Autodesk Inventor part; units mm, degrees
(part 5 of 18)
  spline S48 degree 3 poles (-10072.1223, -10008.9292) (-10072.1359, -10008.9311) (-10072.1627, -10008.9349) (-10072.2009, -10008.9472) (-10072.2359, -10008.9639) (-10072.2669, -10008.9851) (-10072.2932, -10009.0101) (-10072.314, -10009.0387) (-10072.326, -10009.0652) (-10072.3319, -10009.0875) (-10072.3344, -10009.1048) (-10072.335, -10009.1227) (-10072.3334, -10009.141) (-10072.3297, -10009.1596) (-10072.3239, -10009.178) (-10072.3161, -10009.1959) (-10072.3033, -10009.2187) (-10072.2831, -10009.2451) (-10072.2535, -10009.2724) (-10072.2194, -10009.2948) (-10072.1818, -10009.3124) (-10072.1549, -10009.3189) (-10072.1414, -10009.3222) knots 0 0 0 0 0.067054 0.132171 0.195214 0.256087 0.314845 0.371833 0.427831 0.455897 0.484265 0.513193 0.542966 0.573892 0.605563 0.637232 0.669027 0.733247 0.798614 0.865047 0.932273 1 1 1 1
  spline S49 degree 3 poles (-10072.1484, -10009.347) (-10072.1552, -10009.3452) (-10072.1688, -10009.3417) (-10072.1951, -10009.331) (-10072.2261, -10009.3129) (-10072.2593, -10009.2847) (-10072.288, -10009.2513) (-10072.3115, -10009.2138) (-10072.3291, -10009.1734) (-10072.3399, -10009.1312) (-10072.3427, -10009.0953) (-10072.3408, -10009.067) (-10072.3371, -10009.0462) (-10072.3313, -10009.0261) (-10072.3234, -10009.0072) (-10072.3137, -10008.9897) (-10072.2986, -10008.9682) (-10072.2756, -10008.9447) (-10072.2429, -10008.9219) (-10072.2064, -10008.9046) (-10072.1671, -10008.8921) (-10072.1397, -10008.8879) (-10072.1259, -10008.8858) knots 0 0 0 0 0.031337 0.062781 0.126297 0.190936 0.256459 0.32232 0.387875 0.452577 0.516183 0.547678 0.57907 0.610325 0.640706 0.670386 0.69965 0.757762 0.816478 0.876441 0.937726 1 1 1 1
  spline S50 degree 3 poles (-10072.0136, -10008.8866) (-10072.0011, -10008.8889) (-10071.9769, -10008.8935) (-10071.9435, -10008.9084) (-10071.9145, -10008.9285) (-10071.8903, -10008.9537) (-10071.8713, -10008.9835) (-10071.8579, -10009.0174) (-10071.8502, -10009.0548) (-10071.8486, -10009.0953) (-10071.8534, -10009.1379) (-10071.8643, -10009.1807) (-10071.8813, -10009.2213) (-10071.9037, -10009.258) (-10071.9309, -10009.2899) (-10071.9573, -10009.312) (-10071.9802, -10009.3264) (-10071.9982, -10009.3354) (-10072.017, -10009.3428) (-10072.03, -10009.3461) (-10072.0365, -10009.3477) knots 0 0 0 0 0.060227 0.117303 0.172542 0.227241 0.282631 0.339845 0.399897 0.463695 0.532058 0.603464 0.673189 0.741116 0.807351 0.872143 0.90418 0.93608 0.967968 1 1 1 1
  spline S51 degree 3 poles (-10072.0296, -10009.3229) (-10072.0263, -10009.3223) (-10072.0197, -10009.3209) (-10072.01, -10009.3183) (-10072.0005, -10009.3153) (-10071.9882, -10009.3107) (-10071.9732, -10009.3038) (-10071.9562, -10009.294) (-10071.9401, -10009.2827) (-10071.9251, -10009.2702) (-10071.911, -10009.2565) (-10071.9026, -10009.2466) (-10071.8984, -10009.2416) knots 0 0 0 0 0.06406 0.127639 0.190828 0.253706 0.37877 0.503307 0.627605 0.751814 0.875967 1 1 1 1
  spline S52 degree 3 poles (-10071.8529, -10009.0281) (-10071.8545, -10009.0246) (-10071.8575, -10009.0175) (-10071.8632, -10009.0076) (-10071.8696, -10008.9982) (-10071.8767, -10008.9895) (-10071.8845, -10008.9813) (-10071.8931, -10008.9738) (-10071.9022, -10008.9668) (-10071.9121, -10008.9605) (-10071.9225, -10008.9547) (-10071.9335, -10008.9495) (-10071.945, -10008.9449) (-10071.9571, -10008.9408) (-10071.9697, -10008.9373) (-10071.9827, -10008.9343) (-10071.9962, -10008.9318) (-10072.0053, -10008.9306) (-10072.01, -10008.93) knots 0 0 0 0 0.059633 0.118254 0.176262 0.234034 0.291919 0.350232 0.409251 0.469215 0.530325 0.592744 0.656603 0.721998 0.789001 0.857656 0.927988 1 1 1 1
  ellipse E575 centre (-10070.5168, -10009.0175) end of major axis (-10070.2676, -10008.9967) minor radius 0.1227 (-10070.4266, -10008.897) -> (-10070.5389, -10008.8963) ccw
  ellipse E576 centre (-10070.5132, -10009.0609) end of major axis (-10070.7623, -10009.0817) minor radius 0.1227 (-10070.423, -10008.9404) -> (-10070.5353, -10008.9397) ccw
  ellipse E577 centre (-10072.1038, -10009.007) end of major axis (-10071.8546, -10008.9862) minor radius 0.1227 (-10072.0136, -10008.8866) -> (-10072.1259, -10008.8858) ccw
  ellipse E578 centre (-10072.1001, -10009.0504) end of major axis (-10072.3493, -10009.0712) minor radius 0.1227 (-10072.01, -10008.93) -> (-10072.1223, -10008.9292) ccw
  ellipse E579 centre (-10070.5162, -10009.1216) end of major axis (-10070.2755, -10009.1894) minor radius 0.2142 (-10070.5544, -10009.3326) -> (-10070.4426, -10009.3334) ccw
  ellipse E580 centre (-10072.1031, -10009.1112) end of major axis (-10071.8625, -10009.1789) minor radius 0.2142 (-10072.1414, -10009.3222) -> (-10072.0296, -10009.3229) ccw
  ellipse E581 centre (-10070.2084, -10009.1917) end of major axis (-10070.2065, -10008.9037) minor radius 0.0453 (-10070.2293, -10008.9417) -> (-10070.2487, -10009.3347) ccw
  ellipse E582 centre (-10070.2084, -10009.1917) end of major axis (-10070.2107, -10009.5297) minor radius 0.0531 (-10070.2329, -10008.8983) -> (-10070.2557, -10009.3595) ccw
  ellipse E583 centre (-10072.2951, -10009.178) end of major axis (-10072.2973, -10009.516) minor radius 0.0531 (-10072.3196, -10008.8846) -> (-10072.3423, -10009.3457) ccw
  line L687 (-10070.1881, -10008.7391) -> (-10070.2329, -10008.8983)
  line L688 (-10072.3196, -10008.8846) -> (-10072.3149, -10008.8679)
  line L689 (-10072.3105, -10008.8522) -> (-10072.3069, -10008.8393)
  line L690 (-10070.1841, -10008.7811) -> (-10070.2293, -10008.9417)
  line L691 (-10072.2871, -10029.6576) -> (-10072.2821, -10029.5511)
  ellipse E584 centre (-10072.6143, -10008.6378) end of major axis (-10072.3161, -10008.7222) minor radius 0.2558 (-10072.3088, -10008.6455) -> (-10072.3104, -10008.6316) ccw
  line L692 (-10072.3104, -10008.6316) -> (-10072.2913, -10008.5643)
  line L693 (-10072.3046, -10008.6951) -> (-10072.3088, -10008.6455)
  arc A6 (-10072.145, -10030.9182) -> (-10072.0351, -10030.8171) centre (-10072.2938, -10030.6462) ccw
  ellipse E585 centre (-10072.1984, -10008.6427) end of major axis (-10072.1761, -10008.2008) minor radius 0.0791 (-10072.2594, -10008.4435) -> (-10072.261, -10008.4555) ccw
  arc A7 (-10072.0403, -10007.364) -> (-10072.1626, -10007.2386) centre (-10072.3143, -10007.509) ccw
  ellipse E586 centre (-10072.6346, -10029.3671) end of major axis (-10072.3396, -10029.2718) minor radius 0.274 (-10072.3299, -10029.3798) -> (-10072.3284, -10029.365) ccw
  line L694 (-10072.325, -10029.3952) -> (-10072.3299, -10029.3798)
  line L695 (-10072.3284, -10029.365) -> (-10072.3184, -10029.2255)
  ellipse E587 centre (-10072.6677, -10009.4402) end of major axis (-10072.3588, -10009.4144) minor radius 0.1522 (-10072.3645, -10009.4509) -> (-10072.3616, -10009.4422) ccw
  line L696 (-10072.3562, -10009.5506) -> (-10072.3645, -10009.4509)
  ellipse E588 centre (-10072.6401, -10008.8765) end of major axis (-10072.3417, -10008.9605) minor radius 0.2656 (-10072.3339, -10008.8785) -> (-10072.3356, -10008.8642) ccw
  line L697 (-10072.3356, -10008.8642) -> (-10072.3215, -10008.8144)
  line L698 (-10072.3296, -10008.93) -> (-10072.3339, -10008.8785)
  line L699 (-10072.3616, -10009.4422) -> (-10072.3467, -10009.3895)
  ellipse E589 centre (-10072.2686, -10009.2994) end of major axis (-10072.2657, -10008.8569) minor radius 0.0696 (-10072.3276, -10009.0793) -> (-10072.3299, -10009.1054) ccw
  arc A8 (-10070.2041, -10029.4572) -> (-10070.1804, -10029.5914) centre (-10069.8944, -10029.4717) ccw
  line L700 (-10070.1804, -10029.5914) -> (-10070.1612, -10029.6371)
  line L701 (-10070.1889, -10029.1314) -> (-10070.2041, -10029.4572)
  arc A9 (-10070.1531, -10029.8637) -> (-10070.147, -10029.8789) centre (-10069.8629, -10029.7549) ccw
  arc A10 (-10070.1727, -10029.7444) -> (-10070.1621, -10029.8358) centre (-10069.8629, -10029.7549) ccw
  line L702 (-10070.147, -10029.8789) -> (-10070.1076, -10029.9691)
  line L703 (-10070.1685, -10029.6198) -> (-10070.1727, -10029.7444)
  arc A11 (-10064.8037, -10028.4984) -> (-10064.8044, -10028.4963) centre (-10065.9342, -10028.9009) ccw
  line L704 (-10065.7396, -10009.9143) -> (-10064.7957, -10009.8155)
  line L705 (-10065.7396, -10028.2797) -> (-10064.7957, -10028.3785)
  arc A12 (-10064.8044, -10009.6977) -> (-10064.8037, -10009.6956) centre (-10065.9342, -10009.2931) ccw
  arc A13 (-10061.9634, -10012.6939) -> (-10061.989, -10012.5783) centre (-10063.1464, -10012.895) ccw
  line L706 (-10063.2547, -10012.3915) -> (-10063.1965, -10012.3786)
  arc A14 (-10061.989, -10025.6156) -> (-10061.9634, -10025.5) centre (-10063.1464, -10025.299) ccw
  line L707 (-10063.2547, -10025.8025) -> (-10063.1965, -10025.8154)
  arc A15 (-10062.9803, -10029.3632) -> (-10062.946, -10028.8732) centre (-10064.1349, -10029.0362) ccw
  line L708 (-10075.6049, -10030.1318) -> (-10075.4175, -10030.1223)
  line L709 (-10074.3953, -10030.0706) -> (-10074.2526, -10030.0634)
  line L710 (-10068.1084, -10029.7528) -> (-10065.7939, -10029.6358)
  line L711 (-10064.718, -10029.5814) -> (-10064.0364, -10029.5469)
  arc A16 (-10062.0783, -10026.4492) -> (-10062.0721, -10026.3309) centre (-10063.2721, -10026.3271) ccw
  line L712 (-10063.2578, -10025.8122) -> (-10063.1965, -10025.8154)
  line L713 (-10064.0581, -10026.8015) -> (-10063.1016, -10026.8518)
  line L714 (-10064.2047, -10013.5891) -> (-10064.1279, -10013.5729)
  arc A17 (-10061.7588, -10010.2049) -> (-10061.7925, -10009.906) centre (-10062.9587, -10010.1889) ccw
  line L715 (-10063.7731, -10009.7624) -> (-10062.8324, -10009.6564)
  line L716 (-10063.6658, -10010.7869) -> (-10062.717, -10010.6799)
  arc A18 (-10061.7925, -10028.288) -> (-10061.7588, -10027.9891) centre (-10062.9587, -10028.0051) ccw
  line L717 (-10063.6658, -10027.4071) -> (-10062.717, -10027.5141)
  line L718 (-10063.7731, -10028.4315) -> (-10062.8324, -10028.5376)
  line L719 (-10064.2047, -10024.6048) -> (-10064.1279, -10024.6211)
  arc A19 (-10062.0721, -10011.8631) -> (-10062.0783, -10011.7448) centre (-10063.2721, -10011.8669) ccw
  line L720 (-10064.0581, -10011.3925) -> (-10063.1016, -10011.3422)
  line L721 (-10063.2578, -10012.3818) -> (-10063.1965, -10012.3786)
  arc A20 (-10062.946, -10009.3208) -> (-10062.9803, -10008.8308) centre (-10064.1349, -10009.1577) ccw
  line L722 (-10075.6049, -10008.0622) -> (-10075.4175, -10008.0717)
  line L723 (-10074.3953, -10008.1234) -> (-10074.285, -10008.1289)
  line L724 (-10068.1392, -10008.4396) -> (-10065.7939, -10008.5582)
  line L725 (-10064.718, -10008.6126) -> (-10064.0364, -10008.6471)
  line L726 (-10075.5477, -10028.2832) -> (-10075.5066, -10028.2829)
  line L727 (-10068.1881, -10028.2347) -> (-10067.699, -10028.2314)
  line L728 (-10068.3069, -10010.1041) -> (-10066.7715, -10009.9541)
  line L729 (-10068.3069, -10028.0898) -> (-10066.7715, -10028.2399)
  line L730 (-10075.5477, -10009.9108) -> (-10075.5066, -10009.9111)
  line L731 (-10068.1987, -10009.9593) -> (-10067.699, -10009.9625)
  ellipse E590 centre (-10081.3091, -10029.2883) end of major axis (-10081.2663, -10030.9877) minor radius 0.2846 (-10081.484, -10030.4742) -> (-10081.2663, -10030.9877) ccw
  line L732 (-10081.1126, -10030.9839) -> (-10081.2663, -10030.9877)
  ellipse E591 centre (-10081.3091, -10008.9057) end of major axis (-10081.2663, -10007.2062) minor radius 0.2846 (-10081.2663, -10007.2062) -> (-10081.484, -10007.7198) ccw
  line L733 (-10081.1126, -10007.2101) -> (-10081.2663, -10007.2062)
  ellipse E592 centre (-10079.4642, -10029.8112) end of major axis (-10079.3783, -10031.5091) minor radius 0.3038 (-10079.6701, -10030.7592) -> (-10079.3783, -10031.5091) ccw
  line L734 (-10079.235, -10031.5018) -> (-10079.3783, -10031.5091)
  ellipse E593 centre (-10079.4642, -10008.3827) end of major axis (-10079.3783, -10006.6849) minor radius 0.3038 (-10079.3783, -10006.6849) -> (-10079.6701, -10007.4347) ccw
  line L735 (-10079.235, -10006.6922) -> (-10079.3783, -10006.6849)
  ellipse E594 centre (-10082.3808, -10011.9965) end of major axis (-10082.5461, -10010.3045) minor radius 0.0977 (-10082.5461, -10010.3045) -> (-10082.5658, -10010.8219) ccw
  line L736 (-10082.2965, -10010.2801) -> (-10082.5461, -10010.3045)
  ellipse E595 centre (-10082.3808, -10026.1975) end of major axis (-10082.5461, -10027.8895) minor radius 0.0977 (-10082.5658, -10027.3721) -> (-10082.5461, -10027.8895) ccw
  line L737 (-10082.2965, -10027.9138) -> (-10082.5461, -10027.8895)
  ellipse E596 centre (-10078.2538, -10029.2113) end of major axis (-10078.2916, -10027.7118) minor radius 0.2511 (-10078.4794, -10028.3382) -> (-10078.5076, -10028.9618) ccw
  ellipse E597 centre (-10078.2538, -10029.2113) end of major axis (-10078.3017, -10027.3119) minor radius 0.3181 (-10078.5573, -10028.33) -> (-10078.4913, -10030.2755) ccw
  ellipse E598 centre (-10081.0135, -10029.2808) end of major axis (-10080.9656, -10031.1802) minor radius 0.3181 (-10081.2919, -10029.9827) -> (-10080.9656, -10031.1802) ccw
  line L738 (-10079.587, -10031.1455) -> (-10080.9656, -10031.1802)
  ellipse E599 centre (-10077.332, -10011.646) end of major axis (-10077.5298, -10009.7564) minor radius 0.0812 (-10077.4803, -10009.9145) -> (-10077.5448, -10009.9731) ccw
  ellipse E600 centre (-10080.1142, -10011.9374) end of major axis (-10080.3121, -10010.0477) minor radius 0.0812 (-10080.3277, -10010.1584) -> (-10080.3141, -10010.5589) ccw
  line L739 (-10077.5298, -10009.7564) -> (-10079.4891, -10009.9615)
  ellipse E601 centre (-10077.332, -10026.5479) end of major axis (-10077.5298, -10028.4376) minor radius 0.0812 (-10077.5448, -10028.2209) -> (-10077.4803, -10028.2794) ccw
  ellipse E602 centre (-10080.1142, -10026.2566) end of major axis (-10080.3121, -10028.1463) minor radius 0.0812 (-10080.3141, -10027.635) -> (-10080.3277, -10028.0355) ccw
  line L740 (-10077.5298, -10028.4376) -> (-10079.4891, -10028.2324)
  ellipse E603 centre (-10078.2538, -10008.9827) end of major axis (-10078.2161, -10007.4832) minor radius 0.2511 (-10078.5076, -10009.2322) -> (-10078.4794, -10009.8558) ccw
  ellipse E604 centre (-10078.2538, -10008.9827) end of major axis (-10078.206, -10007.0833) minor radius 0.3181 (-10078.4913, -10007.9185) -> (-10078.5573, -10009.864) ccw
  ellipse E605 centre (-10081.0135, -10008.9132) end of major axis (-10080.9656, -10007.0138) minor radius 0.3181 (-10080.9656, -10007.0138) -> (-10081.2919, -10008.2112) ccw
  line L741 (-10079.587, -10007.0485) -> (-10080.9656, -10007.0138)
  ellipse E606 centre (-10076.418, -10029.6572) end of major axis (-10076.3422, -10031.1553) minor radius 0.2681 (-10076.6199, -10028.3765) -> (-10076.1967, -10030.8476) ccw
  ellipse E607 centre (-10076.418, -10029.6572) end of major axis (-10076.322, -10031.5548) minor radius 0.3396 (-10076.7301, -10028.364) -> (-10076.0944, -10030.8424) ccw
  ellipse E608 centre (-10079.1694, -10029.7963) end of major axis (-10079.0734, -10031.6939) minor radius 0.3396 (-10079.4714, -10030.3117) -> (-10079.0734, -10031.6939) ccw
  line L742 (-10076.322, -10031.5548) -> (-10079.0734, -10031.6939)
  ellipse E609 centre (-10075.3771, -10011.5894) end of major axis (-10075.5901, -10009.7014) minor radius 0.0405 (-10075.5342, -10010.0006) -> (-10075.5778, -10010.0057) ccw
  ellipse E610 centre (-10078.1589, -10011.9031) end of major axis (-10078.3718, -10010.0151) minor radius 0.0405 (-10078.3754, -10010.0645) -> (-10078.3587, -10010.3306) ccw
  line L743 (-10075.5901, -10009.7014) -> (-10077.5315, -10009.9203)
  ellipse E611 centre (-10075.3771, -10026.6046) end of major axis (-10075.5901, -10028.4926) minor radius 0.0405 (-10075.5778, -10028.1883) -> (-10075.5342, -10028.1934) ccw
  ellipse E612 centre (-10078.1589, -10026.2909) end of major axis (-10078.3718, -10028.1789) minor radius 0.0405 (-10078.3587, -10027.8634) -> (-10078.3754, -10028.1295) ccw
  line L744 (-10075.5901, -10028.4926) -> (-10077.5315, -10028.2737)
  ellipse E613 centre (-10076.418, -10008.5368) end of major axis (-10076.3422, -10007.0387) minor radius 0.2681 (-10076.1967, -10007.3464) -> (-10076.6199, -10009.8175) ccw
  ellipse E614 centre (-10076.418, -10008.5368) end of major axis (-10076.322, -10006.6392) minor radius 0.3396 (-10076.0944, -10007.3516) -> (-10076.7301, -10009.8299) ccw
  ellipse E615 centre (-10079.1694, -10008.3977) end of major axis (-10079.0734, -10006.5001) minor radius 0.3396 (-10079.0734, -10006.5001) -> (-10079.4714, -10007.8823) ccw
  line L745 (-10076.322, -10006.6392) -> (-10079.0734, -10006.5001)
  ellipse E616 centre (-10080.128, -10028.8283) end of major axis (-10080.1379, -10027.3284) minor radius 0.2359 (-10080.3524, -10028.3047) -> (-10080.3533, -10028.3219) ccw
  ellipse E617 centre (-10080.128, -10028.8283) end of major axis (-10080.1405, -10026.9284) minor radius 0.2988 (-10080.4183, -10028.2983) -> (-10080.3597, -10029.9686) ccw
  ellipse E618 centre (-10082.8931, -10028.8466) end of major axis (-10082.8806, -10030.7465) minor radius 0.2988 (-10082.9672, -10030.6666) -> (-10082.8806, -10030.7465) ccw
  line L746 (-10081.4225, -10030.7369) -> (-10082.8806, -10030.7465)
  ellipse E619 centre (-10079.3006, -10011.6956) end of major axis (-10079.4853, -10009.8046) minor radius 0.1092 (-10079.4271, -10009.955) -> (-10079.5149, -10010.0756) ccw
  ellipse E620 centre (-10082.0827, -10011.9673) end of major axis (-10082.2674, -10010.0763) minor radius 0.1092 (-10082.2674, -10010.0763) -> (-10082.2832, -10010.7889) ccw
  line L747 (-10079.4853, -10009.8046) -> (-10082.2674, -10010.0763)
  ellipse E621 centre (-10079.3006, -10026.4984) end of major axis (-10079.4853, -10028.3894) minor radius 0.1092 (-10079.5149, -10028.1184) -> (-10079.4271, -10028.2389) ccw
  ellipse E622 centre (-10082.0827, -10026.2266) end of major axis (-10082.2674, -10028.1176) minor radius 0.1092 (-10082.2832, -10027.4051) -> (-10082.2674, -10028.1176) ccw
  line L748 (-10079.4853, -10028.3894) -> (-10082.2674, -10028.1176)
  ellipse E623 centre (-10080.128, -10009.3656) end of major axis (-10080.1181, -10007.8657) minor radius 0.2359 (-10080.3533, -10009.8721) -> (-10080.3524, -10009.8893) ccw
  ellipse E624 centre (-10080.128, -10009.3656) end of major axis (-10080.1155, -10007.4657) minor radius 0.2988 (-10080.3597, -10008.2254) -> (-10080.4183, -10009.8957) ccw
  ellipse E625 centre (-10082.8931, -10009.3474) end of major axis (-10082.8806, -10007.4475) minor radius 0.2988 (-10082.8806, -10007.4475) -> (-10082.9672, -10007.5274) ccw
  line L749 (-10081.4225, -10007.4571) -> (-10082.8806, -10007.4475)
  line L750 (-10073.9162, -10027.8417) -> (-10073.8157, -10027.8253)
  line L751 (-10073.7158, -10027.8089) -> (-10066.4278, -10026.6143)
  line L752 (-10066.0115, -10022.636) -> (-10068.219, -10021.7774)
  line L753 (-10066.0115, -10022.6361) -> (-10066.0115, -10022.636)
  line L754 (-10079.4417, -10027.2636) -> (-10075.8108, -10027.6435)
  line L755 (-10073.921, -10027.8412) -> (-10073.9162, -10027.8417)
  line L756 (-10079.4417, -10027.2637) -> (-10078.7164, -10027.3396)
  line L757 (-10066.019, -10022.708) -> (-10066.0115, -10022.6361)
  line L758 (-10066.4278, -10026.6143) -> (-10066.3836, -10026.1917)
  line L759 (-10066.21, -10024.5333) -> (-10066.0115, -10022.636)
  ellipse E626 centre (-10079.4416, -10027.2638) end of major axis (-10078.9364, -10027.3166) minor radius 0.0001 (-10079.4417, -10027.2637) -> (-10079.6749, -10027.2393) ccw
  ellipse E627 centre (-10079.4416, -10027.2638) end of major axis (-10078.4311, -10027.3695) minor radius 0.0002 (-10079.4417, -10027.2636) -> (-10079.9083, -10027.2148) ccw
  ellipse E628 centre (-10085.9551, -10026.5828) end of major axis (-10086.9656, -10026.4771) minor radius 0.0002 (-10086.4218, -10026.5339) -> (-10086.9656, -10026.4771) ccw
  ellipse E629 centre (-10085.9551, -10026.5828) end of major axis (-10086.4604, -10026.53) minor radius 0.0001 (-10086.1884, -10026.5584) -> (-10086.4604, -10026.53) ccw
  line L760 (-10086.9656, -10026.4771) -> (-10086.9331, -10026.1667)
  line L761 (-10079.6749, -10027.2393) -> (-10086.1884, -10026.5584)
  line L762 (-10079.9083, -10027.2148) -> (-10086.4218, -10026.5339)
  line L763 (-10086.9655, -10026.4773) -> (-10087.0694, -10027.4724)
  line L764 (-10086.5642, -10027.5252) -> (-10087.0694, -10027.4724)
  line L765 (-10086.5642, -10027.5252) -> (-10086.4603, -10026.5301)
  line L766 (-10086.9655, -10026.4773) -> (-10086.4603, -10026.5301)
  line L767 (-10087.0694, -10027.4724) -> (-10087.0694, -10027.4724)
  line L768 (-10086.4603, -10026.5301) -> (-10086.4604, -10026.53)
  line L769 (-10086.9656, -10026.4771) -> (-10086.9655, -10026.4773)
  line L770 (-10080.3702, -10023.097) -> (-10079.694, -10023.097)
  line L771 (-10080.3702, -10015.097) -> (-10079.694, -10015.097)
  line L772 (-10080.3702, -10023.097) -> (-10080.8249, -10023.097)
  line L773 (-10080.3702, -10015.097) -> (-10080.8249, -10015.097)
  line L774 (-10080.8249, -10023.097) -> (-10081.2971, -10023.097)
  line L775 (-10081.2971, -10015.097) -> (-10080.8249, -10015.097)
  line L776 (-10087.224, -10014.7755) -> (-10087.3297, -10015.097)
  line L777 (-10086.8245, -10015.097) -> (-10086.7392, -10014.8376)
  line L778 (-10087.3297, -10023.097) -> (-10087.224, -10023.4185)
  line L779 (-10086.7392, -10023.3563) -> (-10086.8245, -10023.097)
  line L780 (-10066.0115, -10015.558) -> (-10066.0115, -10015.5579)
  line L781 (-10068.219, -10016.4166) -> (-10066.0115, -10015.558)
  line L782 (-10066.4278, -10011.5797) -> (-10073.7158, -10010.3851)
  line L783 (-10073.8157, -10010.3687) -> (-10073.9162, -10010.3523)
  line L784 (-10078.7164, -10010.8544) -> (-10079.4417, -10010.9303)
  line L785 (-10079.4417, -10010.9304) -> (-10075.8108, -10010.5505)
  line L786 (-10073.921, -10010.3528) -> (-10073.9162, -10010.3523)
  line L787 (-10066.0115, -10015.5579) -> (-10066.019, -10015.486)
  line L788 (-10066.0115, -10015.558) -> (-10066.21, -10013.6607)
  line L789 (-10066.3836, -10012.0023) -> (-10066.4278, -10011.5797)
  ellipse E630 centre (-10079.4416, -10010.9302) end of major axis (-10079.9469, -10010.9831) minor radius 0.0001 (-10079.6749, -10010.9547) -> (-10079.4417, -10010.9303) ccw
  ellipse E631 centre (-10079.4416, -10010.9302) end of major axis (-10078.4311, -10010.8245) minor radius 0.0002 (-10079.9083, -10010.9792) -> (-10079.4417, -10010.9304) ccw
  ellipse E632 centre (-10085.9551, -10011.6111) end of major axis (-10086.9656, -10011.7169) minor radius 0.0002 (-10086.9656, -10011.7169) -> (-10086.4218, -10011.6601) ccw
  ellipse E633 centre (-10085.9551, -10011.6111) end of major axis (-10086.4604, -10011.664) minor radius 0.0001 (-10086.4604, -10011.664) -> (-10086.1884, -10011.6356) ccw
  line L790 (-10086.9331, -10012.0273) -> (-10086.9656, -10011.7169)
  line L791 (-10079.6749, -10010.9547) -> (-10086.1884, -10011.6356)
  line L792 (-10086.4218, -10011.6601) -> (-10079.9083, -10010.9792)
  line L793 (-10087.0694, -10010.7216) -> (-10086.9655, -10011.7167)
  line L794 (-10086.4603, -10011.6638) -> (-10086.9655, -10011.7167)
  line L795 (-10086.4603, -10011.6638) -> (-10086.5642, -10010.6688)
  line L796 (-10086.5642, -10010.6688) -> (-10087.0694, -10010.7216)
  line L797 (-10087.0694, -10010.7215) -> (-10087.0694, -10010.7216)
  line L798 (-10086.9655, -10011.7167) -> (-10086.9656, -10011.7169)
  line L799 (-10086.4604, -10011.664) -> (-10086.4603, -10011.6638)
  line L800 (-10067.4438, -10022.0789) -> (-10063.85, -10021.097)
  line L801 (-10063.85, -10017.097) -> (-10067.4438, -10016.1151)
  line L802 (-10063.85, -10021.097) -> (-10063.85, -10017.097)
  line L803 (-10064.1716, -10021.4724) -> (-10062.8067, -10021.097)
  line L804 (-10062.8067, -10017.097) -> (-10064.1622, -10016.7241)
  line L805 (-10062.8067, -10021.097) -> (-10062.8067, -10017.097)
  line L806 (-10064.5388, -10027.4644) -> (-10072.0415, -10028.6015)
  line L807 (-10064.5388, -10027.4644) -> (-10064.5388, -10027.4644)
  line L808 (-10072.0415, -10028.6014) -> (-10064.5388, -10027.4644)
  line L809 (-10072.0415, -10028.6015) -> (-10072.0415, -10028.6014)
  line L810 (-10064.0746, -10023.4914) -> (-10066.0191, -10022.708)
  line L811 (-10064.0746, -10023.4915) -> (-10064.0746, -10023.4914)
  line L812 (-10077.5596, -10027.9567) -> (-10072.0415, -10028.6014)
  line L813 (-10077.5596, -10027.9567) -> (-10072.0415, -10028.6015)
  line L814 (-10064.5388, -10027.4644) -> (-10064.0746, -10023.4915)
  line L815 (-10064.5388, -10027.4644) -> (-10064.0746, -10023.4914)
  ellipse E634 centre (-10077.5596, -10027.9568) end of major axis (-10077.055, -10028.0157) minor radius 0 (-10077.5596, -10027.9567) -> (-10077.7926, -10027.9295) ccw
  ellipse E635 centre (-10077.5596, -10027.9568) end of major axis (-10076.5505, -10028.0747) minor radius 0.0001 (-10077.5596, -10027.9567) -> (-10078.0256, -10027.9023) ccw
  ellipse E636 centre (-10084.0644, -10027.1971) end of major axis (-10085.0736, -10027.0792) minor radius 0.0001 (-10084.5304, -10027.1426) -> (-10085.0736, -10027.0792) ccw
  ellipse E637 centre (-10084.0644, -10027.1971) end of major axis (-10084.569, -10027.1382) minor radius 0 (-10084.2974, -10027.1698) -> (-10084.569, -10027.1382) ccw
  line L816 (-10085.0736, -10027.0792) -> (-10085.0269, -10026.6798)
  line L817 (-10077.7926, -10027.9295) -> (-10084.2974, -10027.1698)
  line L818 (-10078.0256, -10027.9023) -> (-10084.5304, -10027.1426)
  line L819 (-10085.0735, -10027.0793) -> (-10085.1895, -10028.0729)
  line L820 (-10084.6849, -10028.1318) -> (-10085.1895, -10028.0729)
  line L821 (-10084.6849, -10028.1318) -> (-10084.569, -10027.1383)
  line L822 (-10085.0735, -10027.0793) -> (-10084.569, -10027.1383)
  line L823 (-10085.1895, -10028.0729) -> (-10085.1894, -10028.0729)
  line L824 (-10084.569, -10027.1383) -> (-10084.569, -10027.1382)
  line L825 (-10085.0736, -10027.0792) -> (-10085.0735, -10027.0793)
  line L826 (-10065.7457, -10021.097) -> (-10073.0163, -10023.097)
  line L827 (-10065.8046, -10021.097) -> (-10065.7457, -10021.097)
  line L828 (-10073.0752, -10023.097) -> (-10065.8046, -10021.097)
  line L829 (-10073.0163, -10023.097) -> (-10073.0752, -10023.097)
  line L830 (-10073.0163, -10015.097) -> (-10065.7457, -10017.097)
  line L831 (-10073.0752, -10015.097) -> (-10073.0163, -10015.097)
  line L832 (-10065.8046, -10017.097) -> (-10073.0752, -10015.097)
  line L833 (-10065.7457, -10017.097) -> (-10065.8046, -10017.097)
  line L834 (-10078.5935, -10023.097) -> (-10073.0752, -10023.097)
  line L835 (-10078.5935, -10015.097) -> (-10073.0752, -10015.097)
  line L836 (-10065.7457, -10021.097) -> (-10065.7457, -10017.097)
  line L837 (-10065.8046, -10021.097) -> (-10065.8046, -10017.097)
  line L838 (-10078.5935, -10023.097) -> (-10079.0461, -10023.097)
  line L839 (-10078.5935, -10015.097) -> (-10079.0461, -10015.097)
  line L840 (-10079.0461, -10023.097) -> (-10079.694, -10023.097)
  line L841 (-10079.694, -10015.097) -> (-10079.0461, -10015.097)
  line L842 (-10085.4009, -10014.8844) -> (-10085.4788, -10015.097)
  line L843 (-10084.9742, -10015.097) -> (-10084.9183, -10014.9444)
  line L844 (-10085.4788, -10023.097) -> (-10085.4009, -10023.3096)
  line L845 (-10084.9183, -10023.2496) -> (-10084.9742, -10023.097)
  line L846 (-10064.0746, -10014.7026) -> (-10064.0746, -10014.7025)
  line L847 (-10066.0191, -10015.486) -> (-10064.0746, -10014.7026)
  line L848 (-10072.0415, -10009.5925) -> (-10064.5388, -10010.7295)
  line L849 (-10072.0415, -10009.5926) -> (-10072.0415, -10009.5925)
  line L850 (-10064.5388, -10010.7296) -> (-10072.0415, -10009.5926)
  line L851 (-10064.5388, -10010.7295) -> (-10064.5388, -10010.7296)
  line L852 (-10072.0415, -10009.5925) -> (-10077.5596, -10010.2372)
  line L853 (-10077.5596, -10010.2373) -> (-10072.0415, -10009.5926)
  line L854 (-10064.0746, -10014.7025) -> (-10064.5388, -10010.7295)
  line L855 (-10064.0746, -10014.7026) -> (-10064.5388, -10010.7296)
  ellipse E638 centre (-10077.5596, -10010.2372) end of major axis (-10078.0642, -10010.2962) minor radius 0 (-10077.7926, -10010.2645) -> (-10077.5596, -10010.2372) ccw
  ellipse E639 centre (-10077.5596, -10010.2372) end of major axis (-10076.5505, -10010.1193) minor radius 0.0001 (-10078.0256, -10010.2917) -> (-10077.5596, -10010.2373) ccw
  ellipse E640 centre (-10084.0644, -10010.9969) end of major axis (-10085.0736, -10011.1148) minor radius 0.0001 (-10085.0736, -10011.1148) -> (-10084.5304, -10011.0514) ccw
  ellipse E641 centre (-10084.0644, -10010.9969) end of major axis (-10084.569, -10011.0558) minor radius 0 (-10084.569, -10011.0558) -> (-10084.2974, -10011.0241) ccw
  line L856 (-10085.0269, -10011.5142) -> (-10085.0736, -10011.1148)
  line L857 (-10077.7926, -10010.2645) -> (-10084.2974, -10011.0241)
  line L858 (-10084.5304, -10011.0514) -> (-10078.0256, -10010.2917)
  line L859 (-10085.1895, -10010.1211) -> (-10085.0735, -10011.1147)
  line L860 (-10084.569, -10011.0557) -> (-10085.0735, -10011.1147)
  line L861 (-10084.569, -10011.0557) -> (-10084.6849, -10010.0622)
  line L862 (-10084.6849, -10010.0622) -> (-10085.1895, -10010.1211)
  line L863 (-10085.1894, -10010.121) -> (-10085.1895, -10010.1211)
  line L864 (-10085.0735, -10011.1147) -> (-10085.0736, -10011.1148)
  line L865 (-10084.569, -10011.0558) -> (-10084.569, -10011.0557)
  line L866 (-10081.35, -10026.6957) -> (-10079.4405, -10026.8767)
  line L867 (-10081.35, -10026.6957) -> (-10080.6219, -10026.7647)
  ellipse E642 centre (-10081.35, -10026.6957) end of major axis (-10080.8443, -10026.7437) minor radius 0 (-10081.35, -10026.6957) -> (-10081.5835, -10026.6736) ccw
  ellipse E643 centre (-10081.35, -10026.6957) end of major axis (-10080.3385, -10026.7916) minor radius 0.0001 (-10081.35, -10026.6957) -> (-10081.817, -10026.6514) ccw
  ellipse E644 centre (-10087.87, -10026.078) end of major axis (-10088.8814, -10025.9821) minor radius 0.0001 (-10088.337, -10026.0337) -> (-10088.8814, -10025.9821) ccw
  ellipse E645 centre (-10087.87, -10026.078) end of major axis (-10088.3757, -10026.0301) minor radius 0 (-10088.1035, -10026.0558) -> (-10088.3757, -10026.0301) ccw
  line L868 (-10088.8814, -10025.9821) -> (-10088.6653, -10023.7019)
  line L869 (-10081.5835, -10026.6736) -> (-10088.1035, -10026.0558)
  line L870 (-10081.817, -10026.6514) -> (-10088.337, -10026.0337)
  line L871 (-10088.8814, -10025.9822) -> (-10088.9758, -10026.978)
  line L872 (-10088.4701, -10027.0259) -> (-10088.9758, -10026.978)
  line L873 (-10088.4701, -10027.0259) -> (-10088.3757, -10026.0301)
  line L874 (-10088.8814, -10025.9822) -> (-10088.3757, -10026.0301)
  line L875 (-10088.9758, -10026.978) -> (-10088.9758, -10026.9781)
  line L876 (-10088.3757, -10026.0301) -> (-10088.3757, -10026.0301)
  line L877 (-10088.8814, -10025.9821) -> (-10088.8814, -10025.9822)
  line L878 (-10082.1916, -10023.097) -> (-10081.2971, -10023.097)
  line L879 (-10082.1916, -10015.097) -> (-10081.2971, -10015.097)
  line L880 (-10082.1916, -10023.097) -> (-10082.6478, -10023.097)
  line L881 (-10082.1916, -10015.097) -> (-10082.6478, -10015.097)
  line L882 (-10088.8463, -10015.097) -> (-10089.3102, -10015.097)
  line L883 (-10089.3102, -10023.097) -> (-10088.8463, -10023.097)
  line L884 (-10089.3102, -10023.097) -> (-10089.3102, -10015.097)
  line L885 (-10082.6478, -10023.097) -> (-10088.8463, -10023.097)
  line L886 (-10088.8463, -10015.097) -> (-10082.6478, -10015.097)
  line L887 (-10088.9133, -10014.097) -> (-10089.2114, -10015.097)
  line L888 (-10088.7056, -10015.097) -> (-10088.5635, -10014.6202)
  line L889 (-10088.7028, -10014.097) -> (-10088.9133, -10014.097)
  line L890 (-10089.2114, -10023.097) -> (-10088.9133, -10024.097)
  line L891 (-10088.7028, -10024.097) -> (-10088.9133, -10024.097)
  line L892 (-10088.5635, -10023.5738) -> (-10088.7056, -10023.097)
  line L893 (-10080.6219, -10011.4293) -> (-10081.35, -10011.4983)
  line L894 (-10081.35, -10011.4983) -> (-10079.4405, -10011.3173)
  ellipse E646 centre (-10081.35, -10011.4982) end of major axis (-10081.8557, -10011.5462) minor radius 0 (-10081.5835, -10011.5204) -> (-10081.35, -10011.4983) ccw
  ellipse E647 centre (-10081.35, -10011.4982) end of major axis (-10080.3385, -10011.4024) minor radius 0.0001 (-10081.817, -10011.5426) -> (-10081.35, -10011.4983) ccw
  ellipse E648 centre (-10087.87, -10012.116) end of major axis (-10088.8814, -10012.2119) minor radius 0.0001 (-10088.8814, -10012.2119) -> (-10088.337, -10012.1603) ccw
  ellipse E649 centre (-10087.87, -10012.116) end of major axis (-10088.3757, -10012.1639) minor radius 0 (-10088.3757, -10012.1639) -> (-10088.1035, -10012.1382) ccw
  line L895 (-10088.6653, -10014.492) -> (-10088.8814, -10012.2119)
  line L896 (-10081.5835, -10011.5204) -> (-10088.1035, -10012.1382)
  line L897 (-10088.337, -10012.1603) -> (-10081.817, -10011.5426)
  line L898 (-10088.9758, -10011.216) -> (-10088.8814, -10012.2118)
  line L899 (-10088.3757, -10012.1639) -> (-10088.8814, -10012.2118)
  line L900 (-10088.3757, -10012.1639) -> (-10088.4701, -10011.1681)
  line L901 (-10088.4701, -10011.1681) -> (-10088.9758, -10011.216)
  line L902 (-10088.9758, -10011.2159) -> (-10088.9758, -10011.216)
  line L903 (-10088.8814, -10012.2118) -> (-10088.8814, -10012.2119)
  line L904 (-10088.3757, -10012.1639) -> (-10088.3757, -10012.1639)
  line L905 (-10077.6915, -10026.8786) -> (-10077.8903, -10026.8578)
  line L906 (-10077.8904, -10026.8576) -> (-10077.6915, -10026.8784)
  line L907 (-10077.8903, -10026.8578) -> (-10077.8904, -10026.8576)
  line L908 (-10077.7175, -10027.1271) -> (-10077.7174, -10027.1273)
  line L909 (-10077.6915, -10026.8784) -> (-10077.7175, -10027.1271)
  line L910 (-10077.5874, -10025.8839) -> (-10077.7864, -10025.863)
  line L911 (-10077.5614, -10025.6352) -> (-10077.5874, -10025.8839)
  line L912 (-10075.6717, -10025.8331) -> (-10075.6977, -10026.0816)
  line L913 (-10075.6718, -10025.8329) -> (-10075.6717, -10025.8331)
  line L914 (-10075.4989, -10026.1024) -> (-10075.6978, -10026.0816)
  line L915 (-10075.6978, -10026.0816) -> (-10075.6718, -10025.8329)
  line L916 (-10075.4988, -10026.1026) -> (-10075.4989, -10026.1024)
  line L917 (-10075.4988, -10026.1026) -> (-10075.5264, -10026.3668)
  line L918 (-10075.9732, -10027.3098) -> (-10077.7174, -10027.1273)
  line L919 (-10077.8904, -10026.8576) -> (-10077.7864, -10025.863)
  line L920 (-10077.5614, -10025.6352) -> (-10075.6718, -10025.8329)
  line L921 (-10075.8278, -10027.3248) -> (-10077.7175, -10027.1271)
  line L922 (-10075.4989, -10026.1024) -> (-10075.6029, -10027.0969)
  line L923 (-10075.8278, -10027.3248) -> (-10075.8018, -10027.0761)
  line L924 (-10075.8018, -10027.0761) -> (-10075.6029, -10027.0969)
  line L925 (-10077.3885, -10025.9047) -> (-10075.8967, -10026.0607)
  line L926 (-10075.8967, -10026.0607) -> (-10076.0007, -10027.0553)
  line L927 (-10076.0007, -10027.0553) -> (-10077.4926, -10026.8992)
  line L928 (-10077.4926, -10026.8992) -> (-10077.3885, -10025.9047)
  line L929 (-10076.0903, -10026.2179) -> (-10077.2315, -10026.0985)
  line L930 (-10075.8967, -10026.0607) -> (-10076.0903, -10026.2179)
  line L931 (-10077.3885, -10025.9047) -> (-10077.2315, -10026.0985)
  line L932 (-10077.2315, -10026.0985) -> (-10077.2988, -10026.7424)
  line L933 (-10077.4926, -10026.8992) -> (-10077.2988, -10026.7424)
  line L934 (-10077.2988, -10026.7424) -> (-10076.1577, -10026.8618)
  line L935 (-10076.0007, -10027.0553) -> (-10076.1577, -10026.8618)
  line L936 (-10076.1577, -10026.8618) -> (-10076.0903, -10026.2179)
  circle A21 centre (-10076.9551, -10026.4529) radius 0.1
  line L937 (-10076.8097, -10026.6189) -> (-10077.1317, -10026.5852)
  line L938 (-10077.1317, -10026.5852) -> (-10077.1317, -10026.5852)
  line L939 (-10076.8096, -10026.6189) -> (-10077.1317, -10026.5852)
  line L940 (-10076.8096, -10026.6189) -> (-10076.8097, -10026.6189)
  line L941 (-10077.1317, -10026.5852) -> (-10077.1005, -10026.2868)
  line L942 (-10077.1005, -10026.2868) -> (-10076.7784, -10026.3205)
  line L943 (-10076.7784, -10026.3206) -> (-10076.7784, -10026.3205)
  line L944 (-10076.7784, -10026.3205) -> (-10076.8097, -10026.6189)
  line L945 (-10076.7784, -10026.3206) -> (-10076.8096, -10026.6189)
  line L946 (-10067.0644, -10025.4919) -> (-10067.0853, -10025.6909)
  line L947 (-10067.0645, -10025.4917) -> (-10067.0644, -10025.4919)
  line L948 (-10067.0853, -10025.6906) -> (-10067.0645, -10025.4917)
  line L949 (-10067.0853, -10025.6909) -> (-10067.0853, -10025.6906)
  line L950 (-10066.8158, -10025.518) -> (-10067.0644, -10025.4919)
  line L951 (-10066.8159, -10025.5177) -> (-10066.8158, -10025.518)
  line L952 (-10067.0645, -10025.4917) -> (-10066.8159, -10025.5177)
  line L953 (-10068.0591, -10025.3879) -> (-10068.3077, -10025.3619)
  line L954 (-10068.0799, -10025.5866) -> (-10068.0798, -10025.5868)
  line L955 (-10068.0591, -10025.3877) -> (-10068.0799, -10025.5866)
  line L956 (-10068.3077, -10025.3616) -> (-10068.0591, -10025.3877)
  line L957 (-10068.3077, -10025.3619) -> (-10068.3077, -10025.3616)
  line L958 (-10067.0853, -10025.6909) -> (-10068.0798, -10025.5868)
  line L959 (-10066.6181, -10023.6283) -> (-10066.8158, -10025.518)
  line L960 (-10067.0853, -10025.6906) -> (-10068.0799, -10025.5866)
  line L961 (-10068.3077, -10025.3616) -> (-10068.11, -10023.472)
  line L962 (-10066.6182, -10023.628) -> (-10066.8159, -10025.5177)
  line L963 (-10067.8406, -10023.2991) -> (-10066.846, -10023.4031)
  line L964 (-10066.8459, -10023.4033) -> (-10066.8667, -10023.602)
  line L965 (-10066.6182, -10023.628) -> (-10066.8668, -10023.602)
  line L966 (-10066.8668, -10023.602) -> (-10066.846, -10023.4031)
  line L967 (-10066.846, -10023.4031) -> (-10066.8459, -10023.4033)
  line L968 (-10066.6181, -10023.6283) -> (-10066.6182, -10023.628)
  line L969 (-10067.8406, -10023.2991) -> (-10067.8614, -10023.498)
  line L970 (-10067.8614, -10023.498) -> (-10068.11, -10023.472)
  line L971 (-10068.0383, -10025.1887) -> (-10067.8822, -10023.6969)
  line L972 (-10067.8822, -10023.6969) -> (-10066.8876, -10023.8009)
  line L973 (-10066.8876, -10023.8009) -> (-10067.0437, -10025.2928)
  line L974 (-10067.0437, -10025.2928) -> (-10068.0383, -10025.1887)
  line L975 (-10067.7251, -10023.8908) -> (-10067.8445, -10025.0319)
  line L976 (-10067.8822, -10023.6969) -> (-10067.7251, -10023.8908)
  line L977 (-10068.0383, -10025.1887) -> (-10067.8445, -10025.0319)
  line L978 (-10067.8445, -10025.0319) -> (-10067.2007, -10025.0992)
  line L979 (-10067.0437, -10025.2928) -> (-10067.2007, -10025.0992)
  line L980 (-10067.2007, -10025.0992) -> (-10067.0813, -10023.9581)
  line L981 (-10066.8876, -10023.8009) -> (-10067.0813, -10023.9581)
  line L982 (-10067.0813, -10023.9581) -> (-10067.7251, -10023.8908)
  circle A22 centre (-10067.4902, -10024.7555) radius 0.1
  line L983 (-10067.3241, -10024.61) -> (-10067.3578, -10024.9321)
  line L984 (-10067.3578, -10024.9321) -> (-10067.3578, -10024.9321)
  line L985 (-10067.3241, -10024.6101) -> (-10067.3578, -10024.9321)
  line L986 (-10067.3241, -10024.6101) -> (-10067.3241, -10024.61)
  line L987 (-10067.3578, -10024.9321) -> (-10067.6562, -10024.9009)
  line L988 (-10067.6562, -10024.9009) -> (-10067.6562, -10024.9009)
  line L989 (-10067.3578, -10024.9321) -> (-10067.6562, -10024.9009)
  line L990 (-10067.6562, -10024.9009) -> (-10067.6225, -10024.5788)
  line L991 (-10067.6225, -10024.5788) -> (-10067.3241, -10024.61)
  line L992 (-10079.0234, -10022.532) -> (-10078.8245, -10022.532)
  line L993 (-10078.8245, -10022.532) -> (-10078.8245, -10022.782)
  line L994 (-10078.8245, -10021.532) -> (-10079.0234, -10021.532)
  line L995 (-10078.8245, -10021.282) -> (-10078.8245, -10021.532)
  line L996 (-10079.0234, -10022.532) -> (-10079.0234, -10021.532)
  line L997 (-10078.8245, -10021.282) -> (-10077.0665, -10021.282)
  line L998 (-10077.0665, -10022.782) -> (-10078.8245, -10022.782)
  line L999 (-10078.6256, -10021.532) -> (-10077.2652, -10021.532)
  line L1000 (-10077.2652, -10022.532) -> (-10078.6256, -10022.532)
  line L1001 (-10078.6256, -10022.532) -> (-10078.6256, -10021.532)
  line L1002 (-10078.6256, -10021.532) -> (-10078.3721, -10021.692)
  line L1003 (-10078.6256, -10022.532) -> (-10078.3721, -10022.372)
  ellipse E650 centre (-10078.0621, -10022.032) end of major axis (-10078.0621, -10021.932) minor radius 0.0995
  ellipse E651 centre (-10078.0569, -10022.032) end of major axis (-10078.0569, -10021.932) minor radius 0.0995 (-10078.0569, -10022.132) -> (-10078.0569, -10021.932) ccw
  line L1004 (-10078.0569, -10022.132) -> (-10078.0621, -10022.132)
  line L1005 (-10078.0569, -10021.932) -> (-10078.0621, -10021.932)
  line L1006 (-10077.8958, -10022.182) -> (-10078.2179, -10022.182)
  line L1007 (-10077.8853, -10022.182) -> (-10077.8958, -10022.182)
  line L1008 (-10078.2179, -10022.182) -> (-10078.2179, -10021.882)
  line L1009 (-10078.2179, -10021.882) -> (-10077.8958, -10021.882)
  line L1010 (-10077.8853, -10021.882) -> (-10077.8958, -10021.882)
  line L1011 (-10077.8958, -10021.882) -> (-10077.8958, -10022.182)
  line L1012 (-10068.4561, -10020.247) -> (-10068.4561, -10020.047)
  line L1013 (-10068.3742, -10020.247) -> (-10068.4561, -10020.247)
  line L1014 (-10068.2074, -10020.047) -> (-10068.1258, -10020.047)
  line L1015 (-10068.4561, -10020.047) -> (-10068.2074, -10020.047)
  line L1016 (-10069.4506, -10020.047) -> (-10069.4506, -10020.247)
  line L1017 (-10069.6993, -10020.047) -> (-10069.4506, -10020.047)
  line L1018 (-10068.4561, -10020.247) -> (-10069.4506, -10020.247)
  line L1019 (-10069.6993, -10020.047) -> (-10069.6993, -10018.147)
  line L1020 (-10068.2074, -10018.147) -> (-10068.2074, -10020.047)
  line L1021 (-10069.4506, -10017.947) -> (-10068.4561, -10017.947)
  line L1022 (-10068.2074, -10018.147) -> (-10068.4561, -10018.147)
  line L1023 (-10068.4561, -10018.147) -> (-10068.4561, -10017.947)
  line L1024 (-10068.4561, -10017.947) -> (-10068.3742, -10017.947)
  line L1025 (-10068.1258, -10018.147) -> (-10068.2074, -10018.147)
  line L1026 (-10069.4506, -10017.947) -> (-10069.4506, -10018.147)
  line L1027 (-10069.4506, -10018.147) -> (-10069.6993, -10018.147)
  line L1028 (-10069.4506, -10019.847) -> (-10069.4506, -10018.347)
  line L1029 (-10069.4506, -10018.347) -> (-10068.4561, -10018.347)
  line L1030 (-10068.4561, -10018.347) -> (-10068.4561, -10019.847)
  line L1031 (-10068.4561, -10019.847) -> (-10069.4506, -10019.847)
  line L1032 (-10069.4506, -10018.347) -> (-10069.2278, -10018.4876)
  line L1033 (-10069.4506, -10019.847) -> (-10069.2278, -10019.7064)
  line L1034 (-10068.4561, -10019.847) -> (-10068.5123, -10019.7079)
  line L1035 (-10068.4561, -10018.347) -> (-10068.5123, -10018.4861)
  ellipse E652 centre (-10068.8753, -10019.3589) end of major axis (-10068.8753, -10019.2589) minor radius 0.0995
  line L1036 (-10068.8708, -10019.4589) -> (-10068.8753, -10019.4589)
  line L1037 (-10068.8708, -10019.2589) -> (-10068.8753, -10019.2589)
  line L1038 (-10066.8667, -10014.5919) -> (-10066.8459, -10014.7906)
  line L1039 (-10066.846, -10014.7909) -> (-10066.8668, -10014.592)
  line L1040 (-10066.8459, -10014.7906) -> (-10066.846, -10014.7909)
  line L1041 (-10066.6182, -10014.5659) -> (-10066.6181, -10014.5657)
  line L1042 (-10066.8668, -10014.592) -> (-10066.6182, -10014.5659)
  line L1043 (-10067.8614, -10014.696) -> (-10067.8406, -10014.8949)
  line L1044 (-10068.11, -10014.722) -> (-10067.8614, -10014.696)
  line L1045 (-10068.3077, -10012.8321) -> (-10068.0591, -10012.8061)
  line L1046 (-10068.3077, -10012.8323) -> (-10068.3077, -10012.8321)
  line L1047 (-10068.0799, -10012.6074) -> (-10068.0591, -10012.8063)
  line L1048 (-10068.0591, -10012.8063) -> (-10068.3077, -10012.8323)
  line L1049 (-10068.0798, -10012.6072) -> (-10068.0799, -10012.6074)
  line L1050 (-10068.0798, -10012.6072) -> (-10067.0853, -10012.5031)
  line L1051 (-10066.8158, -10012.676) -> (-10066.6181, -10014.5657)
  line L1052 (-10066.846, -10014.7909) -> (-10067.8406, -10014.8949)
  line L1053 (-10068.11, -10014.722) -> (-10068.3077, -10012.8323)
  line L1054 (-10066.8159, -10012.6763) -> (-10066.6182, -10014.5659)
  line L1055 (-10068.0799, -10012.6074) -> (-10067.0853, -10012.5034)
  line L1056 (-10067.0853, -10012.5031) -> (-10067.0644, -10012.702)
  line L1057 (-10067.0644, -10012.702) -> (-10066.8158, -10012.676)
  line L1058 (-10066.8159, -10012.6763) -> (-10067.0645, -10012.7023)
  line L1059 (-10067.0645, -10012.7023) -> (-10067.0853, -10012.5034)
  line L1060 (-10067.0853, -10012.5034) -> (-10067.0853, -10012.5031)
  line L1061 (-10067.0645, -10012.7023) -> (-10067.0644, -10012.702)
  line L1062 (-10066.8158, -10012.676) -> (-10066.8159, -10012.6763)
  line L1063 (-10067.8822, -10014.4971) -> (-10068.0383, -10013.0052)
  line L1064 (-10068.0383, -10013.0052) -> (-10067.0437, -10012.9012)
  line L1065 (-10067.0437, -10012.9012) -> (-10066.8876, -10014.393)
  line L1066 (-10066.8876, -10014.393) -> (-10067.8822, -10014.4971)
  line L1067 (-10067.8445, -10013.1621) -> (-10067.7251, -10014.3032)
  line L1068 (-10068.0383, -10013.0052) -> (-10067.8445, -10013.1621)
  line L1069 (-10067.8822, -10014.4971) -> (-10067.7251, -10014.3032)
  line L1070 (-10067.7251, -10014.3032) -> (-10067.0813, -10014.2359)
  line L1071 (-10066.8876, -10014.393) -> (-10067.0813, -10014.2359)
  line L1072 (-10067.0813, -10014.2359) -> (-10067.2007, -10013.0947)
  line L1073 (-10067.0437, -10012.9012) -> (-10067.2007, -10013.0947)
  line L1074 (-10067.2007, -10013.0947) -> (-10067.8445, -10013.1621)
  circle A23 centre (-10067.4357, -10013.9595) radius 0.1
  line L1075 (-10067.3033, -10013.7829) -> (-10067.2696, -10014.1049)
  line L1076 (-10067.2696, -10014.1049) -> (-10067.2696, -10014.1049)
  line L1077 (-10067.3033, -10013.7828) -> (-10067.2696, -10014.1049)
  line L1078 (-10067.3033, -10013.7828) -> (-10067.3033, -10013.7829)
  line L1079 (-10067.2696, -10014.1049) -> (-10067.568, -10014.1361)
  line L1080 (-10067.568, -10014.1361) -> (-10067.6017, -10013.8141)
  line L1081 (-10067.6017, -10013.814) -> (-10067.6017, -10013.8141)
  line L1082 (-10067.6017, -10013.8141) -> (-10067.3033, -10013.7829)
  line L1083 (-10067.6017, -10013.814) -> (-10067.3033, -10013.7828)
  line L1084 (-10064.6, -10020.247) -> (-10064.6, -10020.047)
  line L1085 (-10064.6, -10020.047) -> (-10064.35, -10020.047)
  line L1086 (-10065.6, -10020.047) -> (-10065.6, -10020.247)
  line L1087 (-10065.7457, -10020.047) -> (-10065.6, -10020.047)
  line L1088 (-10064.6, -10020.247) -> (-10065.6, -10020.247)
  line L1089 (-10064.35, -10018.147) -> (-10064.35, -10020.047)
  line L1090 (-10065.6, -10017.947) -> (-10064.6, -10017.947)
  line L1091 (-10064.35, -10018.147) -> (-10064.6, -10018.147)
  line L1092 (-10064.6, -10018.147) -> (-10064.6, -10017.947)
  line L1093 (-10065.6, -10017.947) -> (-10065.6, -10018.147)
  line L1094 (-10065.6, -10018.147) -> (-10065.7457, -10018.147)
  line L1095 (-10065.6, -10019.847) -> (-10065.6, -10018.347)
  line L1096 (-10065.6, -10018.347) -> (-10064.6, -10018.347)
  line L1097 (-10064.6, -10018.347) -> (-10064.6, -10019.847)
  line L1098 (-10064.6, -10019.847) -> (-10065.6, -10019.847)
  line L1099 (-10065.4236, -10018.5233) -> (-10065.4236, -10019.6707)
  line L1100 (-10065.6, -10018.347) -> (-10065.4236, -10018.5233)
  line L1101 (-10065.6, -10019.847) -> (-10065.4236, -10019.6707)
  line L1102 (-10065.4236, -10019.6707) -> (-10064.7763, -10019.6707)
  line L1103 (-10064.6, -10019.847) -> (-10064.7763, -10019.6707)
  line L1104 (-10064.7763, -10019.6707) -> (-10064.7763, -10018.5233)
  line L1105 (-10064.6, -10018.347) -> (-10064.7763, -10018.5233)
  line L1106 (-10064.7763, -10018.5233) -> (-10065.4236, -10018.5233)
  circle A24 centre (-10065.1, -10019.3589) radius 0.1
  line L1107 (-10064.95, -10019.197) -> (-10064.95, -10019.5208)
  line L1108 (-10064.95, -10019.5208) -> (-10065.25, -10019.5208)
  line L1109 (-10065.25, -10019.5208) -> (-10065.25, -10019.197)
  line L1110 (-10065.25, -10019.197) -> (-10064.95, -10019.197)
  line L1111 (-10063.3893, -10020.247) -> (-10063.3893, -10020.047)
  line L1112 (-10063.3893, -10020.047) -> (-10063.141, -10020.047)
  line L1113 (-10063.3893, -10020.247) -> (-10063.85, -10020.247)
  line L1114 (-10063.141, -10018.147) -> (-10063.141, -10020.047)
  line L1115 (-10063.85, -10017.947) -> (-10063.3893, -10017.947)
  line L1116 (-10063.141, -10018.147) -> (-10063.3893, -10018.147)
  line L1117 (-10063.3893, -10018.147) -> (-10063.3893, -10017.947)
  line L1118 (-10063.85, -10018.347) -> (-10063.3893, -10018.347)
  line L1119 (-10063.3893, -10018.347) -> (-10063.3893, -10019.847)
  line L1120 (-10063.3893, -10019.847) -> (-10063.85, -10019.847)
  line L1121 (-10063.85, -10019.6707) -> (-10063.6804, -10019.6707)
  line L1122 (-10063.3893, -10019.847) -> (-10063.6804, -10019.6707)
  line L1123 (-10063.6804, -10019.6707) -> (-10063.6804, -10018.5233)
  line L1124 (-10063.3893, -10018.347) -> (-10063.6804, -10018.5233)
  line L1125 (-10063.6804, -10018.5233) -> (-10063.85, -10018.5233)
  line L1126 (-10063.8297, -10019.197) -> (-10063.8297, -10019.5208)
  line L1127 (-10063.8297, -10019.5208) -> (-10063.85, -10019.5208)
  line L1128 (-10063.85, -10019.197) -> (-10063.8297, -10019.197)
  line L1129 (-10076.0036, -10027.5695) -> (-10075.8049, -10027.5927)
  line L1130 (-10076.0035, -10027.5696) -> (-10076.0036, -10027.5695)
  line L1131 (-10075.8339, -10027.841) -> (-10075.8339, -10027.8412)
  line L1132 (-10075.8049, -10027.5927) -> (-10075.8339, -10027.841)
  line L1133 (-10073.7158, -10027.8089) -> (-10073.719, -10027.8366)
  line L1134 (-10073.9467, -10028.0617) -> (-10075.8339, -10027.8412)
  line L1135 (-10076.0036, -10027.5695) -> (-10075.9732, -10027.3096)
  line L1136 (-10075.5265, -10026.3667) -> (-10073.7727, -10026.5717)
  line L1137 (-10073.9468, -10028.0615) -> (-10075.8339, -10027.841)
  line L1138 (-10073.6031, -10026.8432) -> (-10073.7191, -10027.8364)
  line L1139 (-10073.719, -10027.8366) -> (-10073.8157, -10027.8253)
  line L1140 (-10073.921, -10027.8412) -> (-10073.9467, -10028.0617)
  line L1141 (-10073.9468, -10028.0615) -> (-10073.9178, -10027.8132)
  line L1142 (-10073.9178, -10027.8132) -> (-10073.7191, -10027.8364)